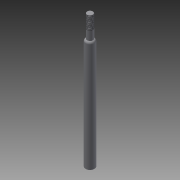
# Autodesk Inventor part: hridel_pro_kola
Saved by Autodesk Inventor 2015 (Build 190159000, 159)
## iProperties
Created: 2012-08-19
Part Number: hridel_pro_kola
Material: Generic
Document SubType Name: Modeling
Designer: idle-rug
Density: 1 g/cm^3
Appearance: Default
Author: idle-rug
Autodesk Inventor part; units mm, degrees
ref_plane "YZ Plane" through (0, 0, 0) normal (1, 0, 0) x (0, 1, 0)
ref_plane "XZ Plane" through (0, 0, 0) normal (0, 1, 0) x (-1, 0, 0)
ref_plane "XY Plane" through (0, 0, 0) normal (0, 0, 1) x (1, 0, 0)
sketch "Sketch1" plane through (0, 0, 0) normal (0, 0, 1) x (1, 0, 0)
  circle A0 centre (0, 0) radius 3
  dimension "d0" = 6
  constraints: 1 centre point, 1 coincident
  measures "d0" diameter of A0
extrude "Extrusion1" add sketch "Sketch1" along normal blind 90
sketch "Sketch2" plane through (0, 0, 90) normal (0, 0, 1) x (1, 0, 0)
  circle A0 centre (0, 0) radius 2
  circle A1 centre (0, 0) radius 3
  dimension "d3" = 4
  constraints: 2 centre point, 2 coincident
  measures "d3" diameter of A0
extrude "Extrusion2" cut sketch "Sketch2" against normal blind 15
thread "Thread1" size "M4x0.7" class "6g" standard "ANSI Metric M Profile" length 10 offset 6
fillet "Fillet1" radius 0.25 1 edges at (-2, 0, 90)
fillet "Fillet2" radius 1.5 1 edges at (-3, 0, 75)
chamfer "Chamfer1" distance 0.5 angle 45 1 edges at (-3, 0, 0)
body "Solid1"
